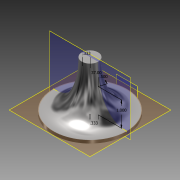
# Autodesk Inventor part: Impeller
Saved by Autodesk Inventor 2018.2 (Build 222227000, 227)
## iProperties
Created: 2018-02-01
Part Number: Impeller
Material: Steel, Galvanized
Document SubType Name: Modeling
Designer: Rus
Density: 7.85 g/cm^3
Appearance: Semi-Polished
Author: Rus
Autodesk Inventor part; units mm, degrees
ref_plane "YZ Plane" through (0, 0, 0) normal (1, 0, 0) x (0, 1, 0)
ref_plane "XZ Plane" through (0, 0, 0) normal (0, 1, 0) x (-1, 0, 0)
ref_plane "XY Plane" through (0, 0, 0) normal (0, 0, 1) x (1, 0, 0)
sketch "Sketch6" plane through (0, 0, 0) normal (0, 1, 0) x (-1, 0, 0)
  circle A0 centre (0, 0) radius 76.2
  dimension "d58" = 152.4
  constraints: 2 coincident, 1 centre point
  measures "d58" diameter of A0
extrude "Extrusion2" add sketch "Sketch6" along normal blind 6.35
sketch "Sketch11" plane through (0, 6.35, 0) normal (0, 1, 0) x (1, 0, 0)
  point P0 (0, 0)
body "Solid2"
